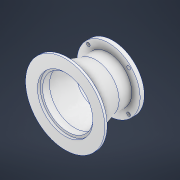
# Autodesk Inventor part: 014
Saved by Autodesk Inventor 2022 (Build 260153000, 153)
## iProperties
Created: 2021-12-31
Part Number: 014
Material: Aluminum 6061
Document SubType Name: Modeling
Designer: vinicius.miguel
Density: 2.7 g/cm^3
Appearance: Aluminum - Flat
Author: vinicius.miguel
Autodesk Inventor part; units mm, degrees
ref_plane "YZ Plane" through (0, 0, 0) normal (1, 0, 0) x (0, 1, 0)
ref_plane "XZ Plane" through (0, 0, 0) normal (0, 1, 0) x (-1, 0, 0)
ref_plane "XY Plane" through (0, 0, 0) normal (0, 0, 1) x (1, 0, 0)
sketch "Sketch1" plane through (0, 0, 0) normal (1, 0, 0) x (0, 1, 0)
  line L0 (0, 0) -> (0, 55.5774) construction
  line L1 (18, -2) -> (18, 16)
  line L2 (23.9, 42.5) -> (26.15, 42.5)
  line L3 (26.15, 42.5) -> (26.15, 45)
  line L4 (26.15, 45) -> (37.5, 45)
  line L5 (37.5, 45) -> (37.5, 42.767)
  line L6 (37.5, 42.767) -> (29.6625, 39.9)
  line L7 (27.9, 35.9) -> (22, 16)
  line L8 (22, 4) -> (29.9, 4)
  line L9 (29.9, 4) -> (29.9, 0)
  line L10 (29.9, 0) -> (20, 0)
  line L11 (20, 0) -> (20, -2)
  line L12 (20, -2) -> (18, -2)
  line L13 (22, 4) -> (22, 16)
  line L14 (29.6625, 39.9) -> (27.9, 39.9)
  line L15 (27.9, 39.9) -> (27.9, 35.9)
  line L16 (23.9, 42.5) -> (23.9, 35.9)
  line L17 (18, 16) -> (23.9, 35.9)
  dimension "d0" = 40
  dimension "d1" = 2
  dimension "d2" = 2
  dimension "d4" = 59.8
  dimension "d5" = 4
  dimension "d7" = 12
  dimension "d8" = 4
  dimension "d9" = 75
  dimension "d10" = 2.233
  dimension "d11" = 52.3
  dimension "d12" = 47.8
  dimension "d13" = 59.325
  dimension "d14" = 5.1
  dimension "d15" = 2.5
  dimension "d16" = 4
  dimension "d17" = 45
  constraints: 36 end point, 9 perpendicular, 4 vertical, 3 horizontal alignment, 2 horizontal, 1 parallel
  measures "d0" diameter of L11 L0
  measures "d1" distance of L10.end L11.end
  measures "d2" distance of L11.end L1.start
  measures "d4" diameter of L9 L0
  measures "d5" distance of L8.end L9.end
  measures "d7" distance of L8.start L7.end
  measures "d8" distance between parallel lines of L1 L13
  measures "d9" diameter of L4.end L0
  measures "d10" distance of L4.end L5.end
  measures "d11" diameter of L3 L0
  measures "d12" diameter of L2.start L0
  measures "d13" diameter of L6.end L0
  measures "d14" distance between parallel lines of L14 L4
  measures "d15" distance of L2.end L3.end
  measures "d16" distance of L14.end L7.start
  measures "d17" distance between parallel lines of L4 L10
revolve "Revolution1" add sketch "Sketch1" angle 360 about axis through (0, 0, 0) along (0, 0, 1)
sketch "Sketch2" plane through (0, 0, 4) normal (0, 0, 1) x (1, 0, 0)
  line L0 (-19.0919, 19.0919) -> (19.0919, 19.0919)
  line L1 (19.0919, 19.0919) -> (19.0919, -19.0919)
  line L2 (19.0919, -19.0919) -> (-19.0919, -19.0919)
  line L3 (-19.0919, -19.0919) -> (-19.0919, 19.0919)
  line L4 (-19.0919, 19.0919) -> (19.0919, -19.0919) construction
  line L5 (19.0919, 19.0919) -> (-19.0919, -19.0919) construction
  point P0 (0, 0)
  dimension "d19" = 54
  constraints: 12 end point, 4 coincident, 2 midpoint, 2 parallel, 2 perpendicular, 1 horizontal
  measures "d19" distance of L0.start L1.end
hole "Hole1" at (-19.0919, 19.0919, 4) at (19.0919, 19.0919, 4) at (-19.0919, -19.0919, 4) at (19.0919, -19.0919, 4) direction (0, 0, -1) diameter 3.4 end through all clearance for "Countersunk Flat Head Screw DIN EN ISO 2009" size "M3" standard "DIN"
body "Solid1"
